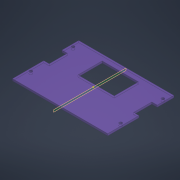
# Autodesk Inventor part: top
Saved by Autodesk Inventor 2022 (Build 260153000, 153)
## iProperties
Created: 2022-01-27
Part Number: top
Material: エポキシ樹脂
Document SubType Name: Modeling
Designer: shiokaze
Density: 1.14 g/cm^3
Appearance: 透明 - スレート 青
Mass: 6.50282 g
Surface Area: 77.9486 cm^2
Volume: 5.70423 cm^3
Author: shiokaze
Autodesk Inventor part; units mm, degrees
ref_plane "YZ Plane" through (0, 0, 0) normal (1, 0, 0) x (0, 1, 0)
ref_plane "XZ Plane" through (0, 0, 0) normal (0, 1, 0) x (-1, 0, 0)
ref_plane "XY Plane" through (0, 0, 0) normal (0, 0, 1) x (1, 0, 0)
sketch "スケッチ1" plane through (0, 0, 0) normal (0, 1, 0) x (-1, 0, 0)
  line L0 (39.4, -27.4) -> (0, -27.4)
  line L1 (0, -27.4) -> (0, 27.4)
  line L2 (0, 27.4) -> (39.4, 27.4)
  line L3 (39.4, -13.5) -> (34.9, -13.5)
  line L4 (34.9, -13.5) -> (34.9, 1.5)
  line L5 (34.9, 1.5) -> (39.4, 1.5)
  line L6 (39.4, 1.5) -> (39.4, -13.5) construction
  line L7 (39.4, 27.4) -> (39.4, 1.5)
  line L8 (39.4, -13.5) -> (39.4, -27.4)
  line L9 (0, -22.4) -> (15, -22.4)
  line L10 (15, -22.4) -> (15, -2.4)
  line L11 (15, -2.4) -> (0, -2.4)
  line L12 (-39.4, -27.4) -> (0, -27.4)
  line L13 (0, 27.4) -> (-39.4, 27.4)
  line L14 (-39.4, -13.5) -> (-34.9, -13.5)
  line L15 (-34.9, -13.5) -> (-34.9, 1.5)
  line L16 (-34.9, 1.5) -> (-39.4, 1.5)
  line L17 (-39.4, 1.5) -> (-39.4, -13.5) construction
  line L18 (-39.4, 27.4) -> (-39.4, 1.5)
  line L19 (-39.4, -13.5) -> (-39.4, -27.4)
  line L20 (0, -22.4) -> (-15, -22.4)
  line L21 (-15, -22.4) -> (-15, -2.4)
  line L22 (-15, -2.4) -> (0, -2.4)
  point P0 (0, 0)
  point P1 (0, 0)
  point P2 (0, 0)
  dimension "d0" = 13.9
  dimension "d1" = 25.9
  dimension "d2" = 39.4
  dimension "d3" = 15
  dimension "d4" = 4.5
  dimension "d5" = 20
  dimension "d6" = 15
  dimension "d7" = 5
  constraints: 46 end point, 8 symmetric about line, 5 parallel, 4 perpendicular, 3 horizontal, 2 coincident, 2 collinear, 2 point on line, 1 midpoint
  measures "d0" distance between parallel lines of L0 L3
  measures "d1" distance between parallel lines of L2 L5
  measures "d2" distance of L1.end L2.end
  measures "d3" distance of L5.end L3.start
  measures "d4" distance between parallel lines of L4 L6
  measures "d5" distance of L9.end L10.end
  measures "d6" distance of L10.end L11.end
  measures "d7" distance between parallel lines of L0 L9
extrude "押し出し1" add sketch "スケッチ1" along normal blind 1.6 contours L0 L1 L9 L10 L11 L2 L7 L5 L4 L3 L8 | L12 L19 L14 L15 L16 L18 L13 L1 L22 L21 L20
sketch "スケッチ2" plane through (0, 1.6, 0) normal (0, 1, 0) x (1, 0, 0)
  line L0 (-39.4, 13.5) -> (-34.9, 13.5) projected
  line L1 (-37.15, 13.5) -> (-37.15, 27.4) construction
  line L2 (-34.9, -1.5) -> (-39.4, -1.5) projected
  line L3 (-37.15, -1.5) -> (-37.15, -27.4) construction
  line L4 (-39.4, -27.4) -> (39.4, -27.4) projected
  line L5 (39.4, 27.4) -> (-39.4, 27.4) projected
  point P0 (0, 0)
  point P1 (-37.15, 20.45)
  point P2 (-37.15, -14.45)
  constraints: 4 end point, 4 midpoint, 2 point on line, 2 vertical
hole "穴1" at (-37.15, 1.6, -20.45) at (-37.15, 1.6, 14.45) direction (0, -1, 0) diameter 2.4 end through all clearance for "Countersunk Flat Head Screw ISO 2009/7046" size "M2" standard "ISO"
ref_plane "作業平面1" through (0, 0, -13.5) normal (-1, 0, 0) x (0, 0, 1)
mirror "ミラー1" about plane through (0, 0, -13.5) normal (-1, 0, 0) of "穴1"
sketch "スケッチ3" plane through (0, 1.6, 0) normal (0, 1, 0) x (1, 0, 0)
  point P0 (0, 0)
